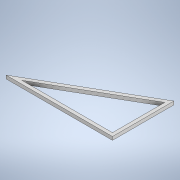
# Autodesk Inventor part: triangle
Saved by Autodesk Inventor 2021.1 (Build 251245010, 245A)
## iProperties
Created: 2020-11-06
Part Number: triangle
Material: Generic
Document SubType Name: Modeling
Designer: robst
Density: 1 g/cm^3
Appearance: Default
Author: robst
Autodesk Inventor part; units mm, degrees
ref_plane "YZ Plane" through (0, 0, 0) normal (1, 0, 0) x (0, 1, 0)
ref_plane "XZ Plane" through (0, 0, 0) normal (0, 1, 0) x (-1, 0, 0)
ref_plane "XY Plane" through (0, 0, 0) normal (0, 0, 1) x (1, 0, 0)
sketch "Sketch1" plane through (0, 0, 0) normal (0, 1, 0) x (-1, 0, 0)
  line L0 (0, 0) -> (0, -117.3176)
  line L1 (0, -117.3176) -> (203.2, 0)
  line L2 (203.2, 0) -> (0, 0)
  line L3 (179.5015, -6.35) -> (6.35, -6.35)
  line L4 (6.35, -6.35) -> (6.35, -106.3191)
  line L5 (6.35, -106.3191) -> (179.5015, -6.35)
  dimension "d0" = 203.2
  dimension "d1" = 30
  dimension "d2" = 6.35
  dimension "d3" = 6.35
  dimension "d4" = 6.35
  constraints: 12 end point, 3 parallel, 1 perpendicular, 1 vertical
  measures "d0" distance of L1.end L0.start
  measures "d1" angle of L1 L2
  measures "d2" distance between parallel lines of L4 L0
  measures "d3" distance between parallel lines of L1 L5
  measures "d4" distance between parallel lines of L3 L2
extrude "Extrusion1" add sketch "Sketch1" along normal blind 6.35
body "Solid1"
